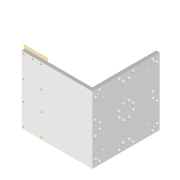
# Autodesk Inventor part: 30_Linear_Captive_Nema8_Stand
Saved by Autodesk Inventor 2022 (Build 260153000, 153)
## iProperties
Created: 2022-12-20
Part Number: 30_Linear_Captive_Nema8_Stand
Material: Generisch
Document SubType Name: Modeling
Designer: diederichbenedict
Density: 1 g/cm^3
Appearance: Vorgabe
Author: diederichbenedict
Autodesk Inventor part; units mm, degrees
ref_plane "YZ Plane" through (0, 0, 0) normal (1, 0, 0) x (0, 1, 0)
ref_plane "XZ Plane" through (0, 0, 0) normal (0, 1, 0) x (-1, 0, 0)
ref_plane "XY Plane" through (0, 0, 0) normal (0, 0, 1) x (1, 0, 0)
ref_plane "Arbeitsebene1" through (0, 0, 0) normal (0, 0, 1) x (1, 0, 0)
sketch "Skizze1" plane through (0, 0, 0) normal (0, 0, 1) x (1, 0, 0)
  circle A0 centre (13.1304, -14.6) radius 1.4 projected
  circle A1 centre (-13.2696, -47) radius 1.4 projected
  circle A2 centre (-13.2696, 47) radius 1.4 projected
  circle A3 centre (13.1304, 14.6) radius 1.4 projected
  circle A4 centre (-0.0696, 47) radius 1.4 projected
  circle A5 centre (-13.2696, 14.6) radius 1.4 projected
  circle A6 centre (13.1304, 47) radius 1.4 projected
  circle A7 centre (13.1304, -47) radius 1.4 projected
  circle A8 centre (-13.2696, -14.6) radius 1.4 projected
  circle A9 centre (0.0304, 14.242) radius 4 projected
  circle A10 centre (0.0304, -10.758) radius 4 projected
  circle A11 centre (0.0304, -35.758) radius 4 projected
  circle A12 centre (0.0304, 39.242) radius 4 projected
  circle A13 centre (0.0304, 1.742) radius 4 projected
  circle A14 centre (0.0304, 26.742) radius 4 projected
  circle A15 centre (0.0304, -23.258) radius 4 projected
  line L0 (16.1304, 50) -> (-16.2696, 50) projected
  line L1 (-16.2696, 50) -> (-16.2696, -50) projected
  line L2 (-16.2696, -50) -> (16.1304, -50) projected
  line L3 (16.1304, -50) -> (16.1304, 50) projected
  line L4 (-16.2696, -50) -> (88.7304, -50)
  line L5 (88.7304, -50) -> (88.7304, 50)
  line L6 (88.7304, 50) -> (-16.2696, 50)
  line L7 (-16.2696, 50) -> (-16.2696, -50)
  point P0 (0, 0)
  dimension "d0" = 105
  dimension "d1" = 100
  constraints: 8 end point, 2 parallel, 1 horizontal, 1 perpendicular
  measures "d0" distance of L6.end L5.end
  measures "d1" distance of L5.end L4.end
extrude "Extrusion1" add sketch "Skizze1" along normal blind 5 contours A9 | A10 | A11 | A12 | A13 | A14 | A15 | L3 L2 L1 L0 | L6 L5 L4 L3
sketch "Skizze2" plane through (-16.2696, -50, 0) normal (0, -1, 0) x (1, 0, 0)
  line L0 (0, 0) -> (105, 0) projected
  line L1 (105, 0) -> (105, 5) projected
  line L2 (0, 5) -> (105, 5) projected
  line L3 (0, 0) -> (0, 5) projected
  line L4 (105, 0) -> (0, 0) projected
  line L5 (105, 0) -> (100, 0)
  line L6 (100, 0) -> (100, -95)
  line L7 (100, -95) -> (105, -95)
  line L8 (105, -95) -> (105, 0)
  point P0 (16.2696, 0)
  dimension "d4" = 5
  dimension "d5" = 95
  constraints: 8 end point, 2 parallel, 1 horizontal, 1 perpendicular
  measures "d4" distance of L7.end L6.end
  measures "d5" distance of L6.end L5.end
extrude "Extrusion2" add sketch "Skizze2" against normal up to surface (100 mm away) contours L0 L8 L7 L6
sketch "Skizze3" plane through (-16.2696, -50, 5) normal (0, -1, 0) x (1, 0, 0)
  line L0 (0, -5) -> (100, -5) projected
  line L1 (100, -5) -> (100, -100) projected
  line L2 (100, -100) -> (105, -100) projected
  line L3 (105, -100) -> (105, 0) projected
  line L4 (0, 0) -> (105, 0) projected
  line L5 (0, -5) -> (0, 0) projected
  line L6 (100, -5) -> (100, -100) projected
  line L7 (100, -100) -> (0, -5)
  point P0 (16.2696, -5)
  constraints: 2 end point
extrude "Extrusion3" add sketch "Skizze3" against normal blind 5 contours L0 L1 L7
sketch "Skizze4" plane through (88.7304, -50, 5) normal (1, 0, 0) x (0, 0, -1)
  line L0 (100, 100) -> (0, 100) projected
  line L1 (0, 0) -> (0, 100) projected
  line L2 (100, 0) -> (0, 0) projected
  line L3 (100, 0) -> (100, 100) projected
  line L4 (92, 92) -> (8, 92)
  line L5 (8, 92) -> (8, 8)
  line L6 (8, 8) -> (92, 8)
  line L7 (92, 8) -> (92, 92)
  line L8 (84, 84) -> (16, 84)
  line L9 (16, 84) -> (16, 16)
  line L10 (16, 16) -> (84, 16)
  line L11 (84, 16) -> (84, 84)
  point P0 (5, 50)
  dimension "d10" = 8
  dimension "d11" = 8
  constraints: 16 end point, 8 coincident, 6 other
  measures "d10" distance between parallel lines of L3 L7
  measures "d11" distance between parallel lines of L7 L11
hole "Bohrung1" at (88.7304, 42, -87) at (88.7304, 34, -79) at (88.7304, -42, -87) at (88.7304, -34, -79) at (88.7304, -34, -11) at (88.7304, -42, -3) at (88.7304, 34, -11) at (88.7304, 42, -3) direction (-1, 0, 0) diameter 2.9 end through all
sketch "Skizze5" plane through (88.7304, -50, 5) normal (1, 0, 0) x (0, 0, -1)
  point P0 (5, 50)
  point P1 (95.8, 89.5)
  point P2 (89.5, 95.8)
  point P3 (60.5, 95.8)
  point P4 (39.5, 95.8)
  point P5 (10.5, 95.8)
  point P6 (4.2, 89.5)
  point P7 (4.2, 60.5)
  point P8 (10.5, 54.2)
  point P9 (39.5, 54.2)
  point P10 (60.5, 54.2)
  point P11 (89.5, 54.2)
  point P12 (89.5, 45.8)
  point P13 (95.8, 39.5)
  point P14 (95.8, 10.5)
  point P15 (89.5, 4.2)
  point P16 (60.5, 4.2)
  point P17 (39.5, 4.2)
  point P18 (10.5, 4.2)
  point P19 (4.2, 10.5)
  point P20 (4.2, 39.5)
  point P21 (10.5, 45.8)
  point P22 (39.5, 45.8)
  point P23 (45.8, 39.5)
  point P24 (54.2, 39.5)
  point P25 (60.5, 45.8)
  point P26 (54.2, 10.5)
  point P27 (45.8, 10.5)
  point P28 (45.8, 89.5)
  point P29 (45.8, 60.5)
  point P30 (54.2, 60.5)
  point P31 (54.2, 89.5)
hole "Bohrung2" at (88.7304, 39.5, -90.8) at (88.7304, 45.8, -84.5) at (88.7304, 45.8, -55.5) at (88.7304, 45.8, -34.5) at (88.7304, 45.8, -5.5) at (88.7304, 39.5, 0.8) at (88.7304, 10.5, 0.8) at (88.7304, 4.2, -5.5) at (88.7304, 4.2, -34.5) at (88.7304, 4.2, -55.5) at (88.7304, 4.2, -84.5) at (88.7304, -4.2, -84.5) at (88.7304, -10.5, -90.8) at (88.7304, -39.5, -90.8) at (88.7304, -45.8, -84.5) at (88.7304, -45.8, -55.5) at (88.7304, -45.8, -34.5) at (88.7304, -45.8, -5.5) at (88.7304, -39.5, 0.8) at (88.7304, -10.5, 0.8) at (88.7304, -4.2, -5.5) at (88.7304, -4.2, -34.5) at (88.7304, -10.5, -40.8) at (88.7304, -10.5, -49.2) at (88.7304, -4.2, -55.5) at (88.7304, -39.5, -49.2) at (88.7304, -39.5, -40.8) at (88.7304, 39.5, -40.8) at (88.7304, 10.5, -40.8) at (88.7304, 10.5, -49.2) at (88.7304, 39.5, -49.2) direction (-1, 0, 0) diameter 4.7 depth 7 tip angle 118
